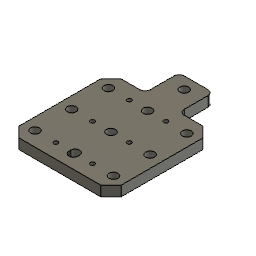
bearing_plate_ed (Autodesk Fusion 360 design; units mm, degrees)
Autodesk Fusion 360 part; units mm, degrees
sketch "Sketch1" plane through (0, 0, 0) normal (0, 1, 0) x (1, 0, 0)
  line L0 (30, 30) -> (30, -30)
  line L1 (30, -30) -> (-30, -30)
  line L2 (-30, -30) -> (-30, 30)
  line L3 (-30, 30) -> (30, -30) construction
  line L4 (30, 30) -> (-30, -30) construction
  line L5 (10, 30) -> (10, 50)
  line L6 (10, 50) -> (-10, 50)
  line L7 (-10, 50) -> (-10, 30)
  line L8 (-30, 30) -> (-10, 30)
  line L9 (10, 30) -> (30, 30)
  circle A0 centre (0, 43) radius 2.6
  line L10 (-30, 0) -> (30, 0) construction
  circle A1 centre (0, 21.5) radius 2.6
  circle A2 centre (-23, 21.5) radius 2.6
  circle A3 centre (23, 21.5) radius 2.6
  circle A4 centre (-10.75, 21.5) radius 1.25
  circle A5 centre (10.75, 21.5) radius 1.25
  circle A6 centre (-23, 0) radius 2.6
  circle A7 centre (-10.75, 0) radius 1.25
  circle A8 centre (0, 0) radius 2.6
  circle A9 centre (10.75, 0) radius 1.25
  circle A10 centre (23, 0) radius 2.6
  circle A11 centre (-23, -21.5) radius 2.6
  circle A12 centre (-10.75, -21.5) radius 1.25
  circle A13 centre (10.75, -21.5) radius 1.25
  circle A14 centre (23, -21.5) radius 2.6
  line L11 (-2.6, -21) -> (-2.6, -22)
  arc A15 (-2.6, -22) -> (2.6, -22) centre (0, -22) ccw
  line L12 (2.6, -22) -> (2.6, -21)
  arc A16 (2.6, -21) -> (-2.6, -21) centre (0, -21) ccw
  point P0 (0, -21.5)
  dimension "d4" = 60
  dimension "d5" = 60
  dimension "d7" = 20
  dimension "d8" = 20
  dimension "d9" = 5.2
  dimension "d10" = 7
  dimension "d11" = 5.2
  dimension "d12" = 21.5
  dimension "d13" = 5.2
  dimension "d14" = 5.2
  dimension "d15" = 23
  dimension "d16" = 23
  dimension "d17" = 2.5
  dimension "d18" = 2.5
  dimension "d19" = 10.75
  dimension "d20" = 10.75
  dimension "d24" = 21.5
  dimension "d25" = 0
  dimension "d28" = 5.2
  dimension "d29" = 0.5
  constraint horizontal L8
  constraint perpendicular L0 L9
  constraint parallel L1 L8
  constraint parallel L0 L2
  constraint coincident L3 A8.centre
  constraint coincident L4 A8.centre
  constraint coincident A8.centre origin
  constraint vertical L5
  constraint horizontal L6
  constraint vertical L7
  constraint collinear L8 L9
  constraint midpoint L2 L10.start
  constraint midpoint L0 L10.end
  constraint tangent L11 A15
  constraint tangent A15 L12
  constraint parallel L11 L12
  constraint tangent L12 A16
  constraint tangent L11 A16
  measures "d4" distance of L0.end L1.end
  measures "d5" distance of L0.start L0.end
  measures "d7" distance of L7.end L5.start
  measures "d8" distance of L7.end L6.end
  measures "d9" diameter of A0
  measures "d10" distance of L6 A0.centre
  measures "d11" diameter of A1
  measures "d12" distance of A0.centre A1.centre
  measures "d13" diameter of A2
  measures "d14" diameter of A3
  measures "d15" distance of A1.centre A2.centre
  measures "d16" distance of A1.centre A3.centre
  measures "d17" diameter of A4
  measures "d18" diameter of A5
  measures "d19" distance of A1.centre A4.centre
  measures "d20" distance of A1.centre A5.centre
  measures "d28" diameter of A15
  measures "d29" distance of A16.centre P0
extrude "Extrude1" add sketch "Sketch1" along normal blind 6
chamfer "Chamfer1" distance 6 angle 45 4 edges at (30, 3, 30) (30, 3, -30) (-30, 3, 30) (-30, 3, -30)
fillet "Fillet1" radius 3 2 edges at (10, 3, -50) (-10, 3, -50)
fillet "Fillet2" radius 3 2 edges at (10, 3, -30) (-10, 3, -30)
equation "larger_hole_radii = 2.6 mm"
equation "small_hole_Radii = 1.25 mm"
equation "base_sqaure_dim = 60 mm"
equation "d4 = base_sqaure_dim"
equation "d5 = base_sqaure_dim"
equation "square_extension = 20 mm"
equation "d7 = square_extension"
equation "d8 = square_extension"
equation "d9 = larger_hole_radii * 2"
equation "d11 = larger_hole_radii * 2"
equation "d13 = 2 * larger_hole_radii"
equation "d14 = 2 * larger_hole_radii"
equation "d17 = small_hole_Radii * 2"
equation "d18 = small_hole_Radii * 2"
equation "dist_between_Rows = 21.50 mm"
equation "slot_height = 5.20 mm"
equation "slot_width = 0.50 mm"
equation "d28 = slot_height"
equation "d29 = slot_width"
equation "ext = 6.0 mm"
equation "d31 = ext"
equation "d33 = ext"
equation "fillet_top = 3 mm"
equation "d36 = fillet_top"
equation "d38 = fillet_top"
